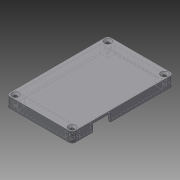
# Autodesk Inventor part: cover
Saved by Autodesk Inventor 2015 (Build 190159000, 159)
## iProperties
Created: 2020-03-18
Part Number: cover
Material: Generic
Document SubType Name: Modeling
Designer: Toby
Density: 1 g/cm^3
Appearance: Default
Author: Toby
Autodesk Inventor part; units mm, degrees
ref_plane "YZ Plane" through (0, 0, 0) normal (1, 0, 0) x (0, 1, 0)
ref_plane "XZ Plane" through (0, 0, 0) normal (0, 1, 0) x (-1, 0, 0)
ref_plane "XY Plane" through (0, 0, 0) normal (0, 0, 1) x (1, 0, 0)
sketch "Sketch1" plane through (0, 0, 0) normal (0, 0, 1) x (1, 0, 0)
  line L0 (-34.1779, 55.6594) -> (21.8221, 55.6594)
  line L1 (21.8221, 55.6594) -> (21.8221, -30.6406)
  line L2 (21.8221, -30.6406) -> (-34.1779, -30.6406)
  line L3 (-34.1779, -30.6406) -> (-34.1779, 55.6594)
  point P0 (0, 0)
  dimension "d0" = 56
  dimension "d1" = 86.3
  constraints: 8 end point, 2 parallel, 1 horizontal, 1 perpendicular
  measures "d0" distance between parallel lines of L1 L3
  measures "d1" distance between parallel lines of L2 L0
extrude "Extrusion1" add sketch "Sketch1" along normal blind 2
sketch "Sketch2" plane through (0, 0, 2) normal (0, 0, 1) x (1, 0, 0)
  line L0 (-34.1779, 55.6594) -> (21.8221, 55.6594)
  line L1 (21.8221, 55.6594) -> (21.8221, -30.6406)
  line L2 (21.8221, -30.6406) -> (-34.1779, -30.6406)
  line L3 (-34.1779, -30.6406) -> (-34.1779, 55.6594)
  line L4 (-32.1779, 53.6594) -> (19.8221, 53.6594)
  line L5 (19.8221, 53.6594) -> (19.8221, -28.6406)
  line L6 (19.8221, -28.6406) -> (-32.1779, -28.6406)
  line L7 (-32.1779, -28.6406) -> (-32.1779, 53.6594)
  point P0 (0, 0)
  dimension "d4" = 2
  dimension "d5" = 2
  dimension "d6" = 2
  dimension "d7" = 2
  constraints: 16 end point, 4 parallel, 2 horizontal, 2 perpendicular
  measures "d4" distance between parallel lines of L4 L0
  measures "d5" distance between parallel lines of L2 L6
  measures "d6" distance between parallel lines of L3 L7
  measures "d7" distance between parallel lines of L1 L5
extrude "Extrusion2" add sketch "Sketch2" along normal blind 14.4
sketch "Sketch3" plane through (0, 0, 2) normal (0, 0, 1) x (1, 0, 0)
  line L0 (-34.1779, 55.6594) -> (-26.1779, 55.6594)
  line L1 (-26.1779, 55.6594) -> (-26.1779, 47.6594)
  line L2 (-26.1779, 47.6594) -> (-34.1779, 47.6594)
  line L3 (-34.1779, 47.6594) -> (-34.1779, 55.6594)
  line L4 (21.8221, 55.6594) -> (13.8221, 55.6594)
  line L5 (13.8221, 55.6594) -> (13.8221, 47.6594)
  line L6 (13.8221, 47.6594) -> (21.8221, 47.6594)
  line L7 (21.8221, 47.6594) -> (21.8221, 55.6594)
  line L8 (-34.1779, -30.6406) -> (-26.1779, -30.6406)
  line L9 (-26.1779, -30.6406) -> (-26.1779, -22.6406)
  line L10 (-26.1779, -22.6406) -> (-34.1779, -22.6406)
  line L11 (-34.1779, -22.6406) -> (-34.1779, -30.6406)
  line L12 (21.8221, -30.6406) -> (13.8221, -30.6406)
  line L13 (13.8221, -30.6406) -> (13.8221, -22.6406)
  line L14 (13.8221, -22.6406) -> (21.8221, -22.6406)
  line L15 (21.8221, -22.6406) -> (21.8221, -30.6406)
  line L16 (-34.1779, -30.6406) -> (21.8221, -30.6406) projected
  point P0 (0, 0)
  dimension "d10" = 8
  dimension "d11" = 8
  dimension "d12" = 8
  dimension "d13" = 8
  dimension "d14" = 8
  dimension "d15" = 8
  dimension "d16" = 8
  dimension "d17" = 8
  constraints: 32 end point, 8 parallel, 4 horizontal, 4 perpendicular, 1 collinear, 1 point on line
  measures "d10" distance of L1.end L2.end
  measures "d11" distance of L0.end L1.end
  measures "d12" distance of L6.end L5.end
  measures "d13" distance of L5.end L4.end
  measures "d14" distance of L10.end L9.end
  measures "d15" distance of L9.end L8.end
  measures "d16" distance of L13.end L14.end
  measures "d17" distance of L12.end L13.end
extrude "Extrusion3" add sketch "Sketch3" along normal blind 14.4
sketch "Sketch4" plane through (0, 0, 16.4) normal (0, 0, 1) x (1, 0, 0)
  line L0 (-26.1779, -22.6406) -> (-32.1779, -22.6406) projected
  line L1 (19.8221, -22.6406) -> (13.8221, -22.6406) projected
  line L2 (21.8221, 55.6594) -> (21.8221, -30.6406) projected
  line L3 (21.8221, 55.6594) -> (-34.1779, 55.6594) projected
  line L4 (-34.1779, -30.6406) -> (-34.1779, 55.6594) projected
  point P0 (0, 0)
  point P1 (-30.1779, 51.6594)
  point P2 (17.8221, 51.6594)
  point P3 (-30.5754, -26.6406)
  point P4 (17.8221, -26.6406)
  dimension "d20" = 4
  dimension "d21" = 4
  dimension "d22" = 4
  dimension "d23" = 4
  dimension "d24" = 4
  dimension "d25" = 4
  dimension "d26" = 4
  measures "d20" distance from line of L0 point (-30.575, -26.641)
  measures "d21" distance from line of L1 point (17.822, -26.641)
  measures "d22" distance from line of L2 point (17.822, -26.641)
  measures "d23" distance from line of L3 point (-30.178, 51.659)
  measures "d24" distance from line of L4 point (-30.178, 51.659)
  measures "d25" distance from line of L3 point (17.822, 51.659)
  measures "d26" distance from line of L2 point (17.822, 51.659)
hole "Hole1" at (-30.1779, 51.6594, 16.4) at (17.8221, 51.6594, 16.4) at (-30.5754, -26.6406, 16.4) at (17.8221, -26.6406, 16.4) direction (0, 0, -1) diameter 3 depth 6 tip angle 118
fillet "Fillet1" radius 3 4 edges at (-34.1779, 55.6594, 8.2) (21.8221, 55.6594, 8.2) (-34.1779, -30.6406, 8.2) (21.8221, -30.6406, 8.2)
sketch "Sketch5" plane through (0, 0, 2) normal (0, 0, 1) x (1, 0, 0)
  line L0 (-32.1779, 47.6594) -> (19.8221, 47.6594)
  line L1 (19.8221, 47.6594) -> (19.8221, 43.3594)
  line L2 (19.8221, 43.3594) -> (-32.1779, 43.3594)
  line L3 (-32.1779, 43.3594) -> (-32.1779, 47.6594)
  line L4 (19.8221, 47.6594) -> (19.8221, -22.6406) projected
  line L5 (-32.1779, -22.6406) -> (19.8221, -22.6406)
  line L6 (19.8221, -22.6406) -> (19.8221, -18.3406)
  line L7 (19.8221, -18.3406) -> (-32.1779, -18.3406)
  line L8 (-32.1779, -18.3406) -> (-32.1779, -22.6406)
  point P0 (0, 0)
  dimension "d35" = 4.3
  dimension "d36" = 4.3
  constraints: 16 end point, 4 parallel, 2 horizontal, 2 perpendicular, 1 collinear, 1 point on line
  measures "d35" distance between parallel lines of L0 L2
  measures "d36" distance between parallel lines of L5 L7
extrude "Extrusion4" add sketch "Sketch5" along normal blind 2.5
sketch "Sketch6" plane through (0, 0, 16.4) normal (0, 0, 1) x (1, 0, 0)
  line L0 (-34.1779, 55.6594) -> (21.8221, 55.6594)
  line L1 (21.8221, 55.6594) -> (21.8221, -30.6406)
  line L2 (21.8221, -30.6406) -> (-34.1779, -30.6406)
  line L3 (-34.1779, -30.6406) -> (-34.1779, 55.6594)
  line L4 (18.8221, 55.6594) -> (-31.1779, 55.6594) projected
  line L5 (-34.1779, 52.6594) -> (-34.1779, -27.6406) projected
  line L6 (21.8221, -27.6406) -> (21.8221, 52.6594) projected
  line L7 (-31.1779, -30.6406) -> (18.8221, -30.6406) projected
  point P0 (0, 0)
  constraints: 8 end point, 4 collinear, 2 parallel, 1 horizontal, 1 perpendicular
extrude "Extrusion5" add sketch "Sketch6" along normal blind 8.5
sketch "Sketch7" plane through (-31.1779, -30.6406, 0) normal (0, -1, 0) x (1, 0, 0)
  line L0 (-3, 16.4) -> (53, 16.4)
  line L1 (53, 16.4) -> (53, 0)
  line L2 (53, 0) -> (-3, 0)
  line L3 (-3, 0) -> (-3, 16.4)
  point P0 (31.1779, 0)
  constraints: 8 end point, 2 parallel, 1 horizontal, 1 perpendicular
extrude "Extrusion6" cut sketch "Sketch7" against normal blind 300
fillet "Fillet2" radius 3 4 edges at (-34.1779, -30.6406, 20.65) (21.8221, -30.6406, 20.65) (-34.1779, 55.6594, 20.65) (21.8221, 55.6594, 20.65)
sketch "Sketch8" plane through (0, 0, 16.4) normal (0, 0, -1) x (-1, 0, 0)
  line L0 (26.1779, -28.6406) -> (-13.8221, -28.6406)
  line L1 (-13.8221, -28.6406) -> (-13.8221, 53.6594)
  line L2 (-13.8221, 53.6594) -> (26.1779, 53.6594)
  line L3 (26.1779, 53.6594) -> (26.1779, -28.6406)
  line L4 (-19.8221, -22.6406) -> (32.1779, -22.6406)
  line L5 (32.1779, -22.6406) -> (32.1779, 47.6594)
  line L6 (32.1779, 47.6594) -> (-19.8221, 47.6594)
  line L7 (-19.8221, 47.6594) -> (-19.8221, -22.6406)
  line L8 (31.1779, -30.6406) -> (-18.8221, -30.6406) projected
  line L9 (-18.8221, 55.6594) -> (31.1779, 55.6594) projected
  line L10 (34.1779, 52.6594) -> (34.1779, -27.6406) projected
  line L11 (-21.8221, -27.6406) -> (-21.8221, 52.6594) projected
  point P0 (0, 0)
  dimension "d44" = 8
  dimension "d45" = 8
  dimension "d46" = 8
  dimension "d47" = 8
  dimension "d48" = 2
  dimension "d49" = 2
  dimension "d50" = 2
  dimension "d51" = 2
  constraints: 16 end point, 4 parallel, 2 horizontal, 2 perpendicular
  measures "d44" distance between parallel lines of L8 L4
  measures "d45" distance between parallel lines of L9 L6
  measures "d46" distance between parallel lines of L10 L3
  measures "d47" distance between parallel lines of L11 L1
  measures "d48" distance between parallel lines of L11 L7
  measures "d49" distance between parallel lines of L8 L0
  measures "d50" distance between parallel lines of L10 L5
  measures "d51" distance between parallel lines of L9 L2
extrude "Extrusion7" cut sketch "Sketch8" against normal blind 6.5
sketch "Sketch9" plane through (0, 0, 24.9) normal (0, 0, 1) x (1, 0, 0)
  line L0 (-34.1779, 52.6594) -> (-34.1779, -27.6406) projected
  line L1 (18.8221, 55.6594) -> (-31.1779, 55.6594) projected
  line L2 (21.8221, -27.6406) -> (21.8221, 52.6594) projected
  line L3 (-31.1779, -30.6406) -> (18.8221, -30.6406) projected
  point P0 (0, 0)
  point P1 (-30.1779, 51.6594)
  point P2 (17.8221, 51.6594)
  point P3 (-30.1779, -26.6406)
  point P4 (17.8221, -26.6406)
  dimension "d54" = 4
  dimension "d55" = 4
  dimension "d56" = 4
  dimension "d57" = 4
  dimension "d58" = 4
  dimension "d59" = 4
  dimension "d60" = 4
  dimension "d61" = 4
  measures "d54" distance from line of L0 point (-30.178, 51.659)
  measures "d55" distance from line of L1 point (-30.178, 51.659)
  measures "d56" distance from line of L1 point (17.822, 51.659)
  measures "d57" distance from line of L2 point (17.822, 51.659)
  measures "d58" distance from line of L3 point (-30.178, -26.641)
  measures "d59" distance from line of L0 point (-30.178, -26.641)
  measures "d60" distance from line of L3 point (17.822, -26.641)
  measures "d61" distance from line of L2 point (17.822, -26.641)
hole "Hole2" at (-30.1779, 51.6594, 24.9) at (17.8221, 51.6594, 24.9) at (-30.1779, -26.6406, 24.9) at (17.8221, -26.6406, 24.9) direction (0, 0, -1) diameter 3 depth 8 tip angle 118 countersink diameter 6 countersink angle 90
sketch "Sketch10" plane through (21.8221, -27.6406, 24.9) normal (1, 0, 0) x (0, 0, -1)
  line L0 (8.5, 5) -> (8.5, 75.3) projected
  line L1 (8.5, 14.5) -> (2, 14.5)
  line L2 (2, 14.5) -> (2, 29.5)
  line L3 (2, 29.5) -> (8.5, 29.5)
  line L4 (8.5, 29.5) -> (8.5, 14.5)
  line L5 (0, -3) -> (8.5, -3) projected
  point P0 (24.9, 27.6406)
  dimension "d69" = 17.5
  dimension "d70" = 32.5
  dimension "d71" = 6.5
  constraints: 8 end point, 2 parallel, 1 horizontal, 1 perpendicular, 1 point on line
  measures "d69" distance between parallel lines of L5 L1
  measures "d70" distance between parallel lines of L5 L3
  measures "d71" distance between parallel lines of L0 L2
extrude "Extrusion8" cut sketch "Sketch10" against normal blind 6.5
sketch "Sketch11" plane through (0, 0, 22.9) normal (0, 0, -1) x (-1, 0, 0)
  line L0 (32.1779, 47.6594) -> (32.1779, -22.6406) projected
  line L1 (-19.8221, -22.6406) -> (32.1779, -22.6406)
  line L2 (32.1779, -22.6406) -> (32.1779, 47.6594)
  line L3 (32.1779, 47.6594) -> (-19.8221, 47.6594)
  line L4 (-19.8221, 47.6594) -> (-19.8221, -22.6406)
  line L5 (-19.8221, 47.6594) -> (-13.8221, 47.6594) projected
  point P0 (0, 0)
  constraints: 8 end point, 2 parallel, 1 collinear, 1 horizontal, 1 perpendicular, 1 point on line
extrude "Extrusion9" cut sketch "Sketch11" against normal blind 0.8
body "Solid1"
